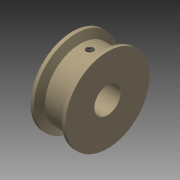
# Autodesk Inventor part: 砂轮电机皮带轮
Saved by Autodesk Inventor 2015 (Build 190159000, 159)
## iProperties
Created: 2017-05-24
Part Number: 砂轮电机皮带轮
Material: 常规
Document SubType Name: Modeling
Designer: Administrator
Density: 1 g/cm^3
Appearance: 麦色
Author: Administrator
Autodesk Inventor part; units mm, degrees
ref_plane "YZ Plane" through (0, 0, 0) normal (1, 0, 0) x (0, 1, 0)
ref_plane "XZ Plane" through (0, 0, 0) normal (0, 1, 0) x (-1, 0, 0)
sketch "草图1" plane through (0, 0, 0) normal (0, 0, 1) x (1, 0, 0)
  line L0 (-10, 0) -> (10, 0)
  line L1 (10, 0) -> (10, 24)
  line L2 (10, 24) -> (8, 24)
  line L3 (8, 24) -> (5.6906, 20)
  line L4 (5.6906, 20) -> (-5.6906, 20)
  line L5 (-5.6906, 20) -> (-8, 24)
  line L6 (-8, 24) -> (-10, 24)
  line L7 (-10, 24) -> (-10, 0)
  line L8 (-14, 0) -> (14, 0) projected
  point P0 (0, 0)
  point P1 (0, 0)
  dimension "d1" = 24
  dimension "d2" = 4
  dimension "d4" = 20
  dimension "d5" = 2
  dimension "d6" = 120
  dimension "d7" = 120
  dimension "d8" = 2
  constraints: 16 end point, 2 parallel, 2 perpendicular, 2 point on line, 1 coincident, 1 horizontal, 1 midpoint
  measures "d1" distance of L0.end L1.end
  measures "d2" distance between parallel lines of L2 L4
  measures "d4" distance of L0.start L0.end
  measures "d5" distance of L5.end L6.end
  measures "d6" angle of L6 L5
  measures "d7" angle of L2 L3
  measures "d8" distance of L1.end L2.end
revolve "旋转1" add sketch "草图1" angle 360 about axis through (-10, 0, 0) along (1, 0, 0)
sketch "草图2" plane through (10, 0, 0) normal (1, 0, 0) x (0, 0, -1)
  circle A0 centre (0, 0) radius 7.5
  dimension "d10" = 15
  constraints: 1 centre point, 1 coincident
  measures "d10" diameter of A0
extrude "拉伸1" cut sketch "草图2" against normal through all
ref_plane "工作平面1" through (0, 0, 20) normal (0, 0, 1) x (1, 0, 0)
sketch "草图3" plane through (0, 0, 20) normal (0, 0, 1) x (1, 0, 0)
  circle A0 centre (0, 0) radius 2
  dimension "d13" = 4
  constraints: 1 centre point, 1 coincident
  measures "d13" diameter of A0
extrude "拉伸2" cut sketch "草图3" against normal up to surface
thread "螺纹1" size "M4x0.7" class "6H" standard "ANSI Metric M Profile" full length
